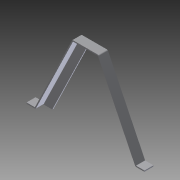
# Autodesk Inventor part: 8 ball lift frame
Saved by Autodesk Inventor 2012 (Build 160160000, 160)
## iProperties
Created: 2013-10-11
Part Number: 8 ball lift frame
Material: Default
Document SubType Name: Modeling
Designer: Bryce
Density: 1 g/cm^3
Author: Bryce
Autodesk Inventor part; units mm, degrees
ref_plane "YZ Plane" through (0, 0, 0) normal (1, 0, 0) x (0, 1, 0)
ref_plane "XZ Plane" through (0, 0, 0) normal (0, 1, 0) x (-1, 0, 0)
ref_plane "XY Plane" through (0, 0, 0) normal (0, 0, 1) x (1, 0, 0)
sketch "Sketch1" plane through (0, 0, 0) normal (0, 0, 1) x (1, 0, 0)
  line L0 (130.175, 215.9) -> (200.025, 215.9)
  line L1 (130.175, 215.9) -> (25.4, 0)
  line L2 (200.025, 215.9) -> (304.8, 0)
  line L3 (306.7883, 3.175) -> (202.0133, 219.075)
  line L4 (202.0133, 219.075) -> (128.1867, 219.075)
  line L5 (128.1867, 219.075) -> (23.4117, 3.175)
  line L6 (25.4, 0) -> (50.1039, 0)
  line L7 (50.1039, 0) -> (154.1085, 214.3125)
  line L8 (172.5624, 214.3125) -> (276.567, 0)
  line L9 (276.567, 0) -> (304.8, 0)
  line L10 (129.4046, 214.3125) -> (154.1085, 214.3125)
  line L11 (172.5624, 214.3125) -> (200.7954, 214.3125)
  line L12 (50.1039, 0) -> (276.567, 0) construction
  line L13 (25.4, 0) -> (0, 0)
  line L14 (0, 0) -> (0, 3.175)
  line L15 (0, 3.175) -> (23.4117, 3.175)
  line L16 (304.8, 0) -> (330.2, 0)
  line L17 (330.2, 0) -> (330.2, 3.175)
  line L18 (330.2, 3.175) -> (306.7883, 3.175)
  dimension "d1" = 69.85
  dimension "d5" = 3.175
  dimension "d34" = 22.225
  dimension "d35" = 25.4
  dimension "d37" = 1.5875
  dimension "d41" = 3.175
  dimension "d43" = 219.075
  dimension "d44" = 3.175
  dimension "d45" = 64.113
  dimension "d46" = 64.113
  dimension "d47" = 3.175
  dimension "d48" = 25.4
  dimension "d49" = 25.4
  dimension "d50" = 330.2
  constraints: 38 end point, 9 parallel, 3 horizontal, 3 point on line, 2 coincident, 2 horizontal alignment, 2 perpendicular, 1 collinear
  measures "d1" distance of L0.start L0.end
  measures "d5" distance between parallel lines of L4 L0
  measures "d34" distance between parallel lines of L7 L1
  measures "d35" distance between parallel lines of L8 L2
  measures "d37" distance between parallel lines of L0 L10
  measures "d41" distance between parallel lines of L5 L1
  measures "d43" distance between parallel lines of L12 L4
  measures "d44" distance between parallel lines of L3 L2
  measures "d45" angle of L12 L7
  measures "d46" angle of L12 L8
  measures "d47" distance of L13.end L14.end
  measures "d48" distance of L1.end L13.end
  measures "d49" distance of L2.end L16.end
  measures "d50" distance between parallel lines of L17 L14
extrude "Extrusion1" add sketch "Sketch1" along normal blind 25.4 contours L1 L13 L14 L15 L5 L4 L3 L18 L17 L16 L2 L0
extrude "Extrusion2" add sketch "Sketch1" along normal blind 3.175
fillet "Fillet1" radius 0.7937 6 edges at (130.175, 215.9, 12.7) (200.025, 215.9, 12.7) (200.7954, 214.3125, 1.5875) (129.4046, 214.3125, 1.5875) (23.4117, 3.175, 12.7) (306.7883, 3.175, 12.7)
fillet "Fillet2" radius 3.175 4 edges at (128.1867, 219.075, 12.7) (202.0133, 219.075, 12.7) (25.4, 0, 14.2875) (304.8, 0, 14.2875)
equation "\"d5\" = d4"
equation "\"d37\" = d36"
equation "\"d44\" = d41"
equation "\"d45\" = d46"
equation "\"d47\" = d41"
equation "\"d49\" = d48"
equation "\"d36\" = 0.5 * d5"
equation "\"d4\" = 3.175"
body "Solid1"
